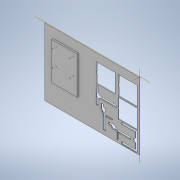
# Autodesk Inventor part: Base
Saved by Autodesk Inventor 2022 (Build 260153000, 153)
## iProperties
Created: 2022-11-21
Part Number: Base
Material: Genérico
Document SubType Name: Modeling
Designer: javie
Density: 1 g/cm^3
Appearance: Valor por defecto
Autodesk Inventor part; units mm, degrees
ref_plane "YZ Plane" through (0, 0, 0) normal (1, 0, 0) x (0, 1, 0)
ref_plane "XZ Plane" through (0, 0, 0) normal (0, 1, 0) x (-1, 0, 0)
ref_plane "XY Plane" through (0, 0, 0) normal (0, 0, 1) x (1, 0, 0)
sketch "Boceto1" plane through (0, 0, 0) normal (0, 0, 1) x (1, 0, 0)
  circle A0 centre (-147.8951, -213.4011) radius 3.5
  circle A1 centre (-21.8951, -213.4011) radius 3.5
  circle A2 centre (-147.8951, -339.4011) radius 3.5
  circle A3 centre (-21.8951, -339.4011) radius 3.5
  circle A4 centre (-309.6354, -191.7984) radius 3.5
  circle A5 centre (-309.6354, -65.7984) radius 3.5
  circle A6 centre (-183.6354, -191.7984) radius 3.5
  circle A7 centre (-183.6354, -65.7984) radius 3.5
  circle A8 centre (-146.8282, -191.7984) radius 3.5
  circle A9 centre (-146.8282, -65.7984) radius 3.5
  circle A10 centre (-20.8282, -191.7984) radius 3.5
  circle A11 centre (-20.8282, -65.7984) radius 3.5
  circle A12 centre (-217.6796, -404.2586) radius 3.5
  circle A13 centre (-276.1451, -313.6219) radius 3.5
  line L0 (-317.237, -262.6146) -> (-317.237, -210.942)
  line L1 (-317.237, -210.942) -> (-302.237, -210.942)
  line L2 (-302.237, -210.942) -> (-302.237, -256.0675)
  circle A14 centre (-309.9844, -222.642) radius 3.5
  line L3 (-29.8951, -324.021) -> (-29.8951, -338.4011)
  line L4 (-29.8951, -338.4011) -> (-139.8951, -338.4011)
  line L5 (-139.8951, -338.4011) -> (-139.8951, -324.4011)
  line L6 (-139.8951, -324.4011) -> (-139.8951, -292.2756)
  arc A15 (-157.9179, -437.9883) -> (-161.9179, -437.9883) centre (-159.9179, -437.9883) ccw
  line L7 (-157.9179, -437.9883) -> (-157.9179, -475.168)
  arc A16 (-161.9179, -475.168) -> (-157.9179, -475.168) centre (-159.9179, -475.168) ccw
  line L8 (-161.9179, -475.168) -> (-161.9179, -437.9883)
  line L9 (-61.4887, -423.9723) -> (-61.4887, -416.4723)
  line L10 (-61.4887, -416.4723) -> (-145.4587, -416.4723)
  arc A17 (-148.1709, -416.0975) -> (-145.4587, -416.4723) centre (-145.4587, -406.4723) ccw
  line L11 (-148.1709, -416.0975) -> (-172.3586, -409.282)
  arc A18 (-172.3586, -409.282) -> (-174.2641, -408.9398) centre (-175.0707, -418.9072) ccw
  arc A19 (-176.1813, -408.5942) -> (-174.2641, -408.9398) centre (-173.4575, -398.9723) ccw
  line L12 (-242.4154, -373.3836) -> (-205.2357, -373.3836)
  arc A20 (-205.2357, -373.3836) -> (-205.2357, -369.3836) centre (-205.2357, -371.3836) ccw
  line L13 (-205.2357, -369.3836) -> (-242.4154, -369.3836)
  arc A21 (-242.4154, -369.3836) -> (-242.4154, -373.3836) centre (-242.4154, -371.3836) ccw
  line L14 (-153.8282, -119.471) -> (-153.8282, -58.7984)
  line L15 (-153.8282, -58.7984) -> (-13.8282, -58.7984)
  line L16 (-13.8282, -58.7984) -> (-13.8282, -198.7984)
  line L17 (-13.8282, -198.7984) -> (-153.8282, -198.7984)
  line L18 (-153.8282, -198.7984) -> (-153.8282, -138.1258)
  line L19 (-138.8282, -144.6729) -> (-138.8282, -183.7984)
  line L20 (-138.8282, -183.7984) -> (-28.8282, -183.7984)
  line L21 (-28.8282, -183.7984) -> (-28.8282, -73.7984)
  line L22 (-28.8282, -73.7984) -> (-138.8282, -73.7984)
  line L23 (-138.8282, -73.7984) -> (-138.8282, -112.9239)
  line L24 (-316.6354, -119.471) -> (-316.6354, -58.7984)
  line L25 (-316.6354, -58.7984) -> (-176.6354, -58.7984)
  line L26 (-176.6354, -58.7984) -> (-176.6354, -198.7984)
  line L27 (-176.6354, -198.7984) -> (-316.6354, -198.7984)
  line L28 (-316.6354, -198.7984) -> (-316.6354, -138.1258)
  line L29 (-301.6354, -144.6729) -> (-301.6354, -183.7984)
  line L30 (-301.6354, -183.7984) -> (-191.6354, -183.7984)
  line L31 (-191.6354, -183.7984) -> (-191.6354, -73.7984)
  line L32 (-191.6354, -73.7984) -> (-301.6354, -73.7984)
  line L33 (-301.6354, -73.7984) -> (-301.6354, -112.9239)
  line L34 (492.5651, -223.6733) -> (492.5651, -502.5112)
  line L35 (492.5651, -502.5112) -> (302.0855, -502.5112)
  line L36 (302.0855, -502.5112) -> (302.0855, -223.6733)
  line L37 (302.0855, -223.6733) -> (492.5651, -223.6733)
  circle A22 centre (459.6774, -256.2358) radius 2.5
  circle A23 centre (459.6774, -382.2358) radius 2.5
  circle A24 centre (333.6774, -256.2358) radius 2.5
  circle A25 centre (333.6774, -382.2358) radius 2.5
  circle A26 centre (-22, -486) radius 3.5
  line L38 (-128.3631, -478) -> (-30, -478)
  line L39 (-30, -478) -> (-30, -438.8745)
  line L40 (-128.3631, -493) -> (-128.3631, -478)
  line L41 (-128.3631, -353) -> (-15, -353)
  line L42 (-15, -353) -> (-15, -413.6726)
  line L43 (-128.3631, -368) -> (-128.3631, -353)
  circle A27 centre (-22, -360) radius 3.5
  arc A28 (-316.6354, -119.471) -> (-316.6354, -138.1258) centre (-303.6354, -128.7984) ccw
  arc A29 (-153.8282, -119.471) -> (-153.8282, -138.1258) centre (-140.8282, -128.7984) ccw
  arc A30 (-317.237, -262.6146) -> (-317.237, -281.2693) centre (-304.237, -271.942) ccw
  arc A31 (-154.8951, -267.0738) -> (-154.8951, -285.7285) centre (-141.8951, -276.4011) ccw
  arc A32 (-281.1451, -332.0528) -> (-271.8095, -355.1202) centre (-267.1529, -339.8128) ccw
  arc A33 (-30, -407.1255) -> (-30, -438.8745) centre (-28, -423) ccw
  arc A34 (-207.2589, -415.9528) -> (-179.6123, -423.9723) centre (-191.4887, -413.2508) ccw
  arc A35 (-301.6354, -144.6729) -> (-301.6354, -112.9239) centre (-303.6354, -128.7984) ccw
  arc A36 (-138.8282, -144.6729) -> (-138.8282, -112.9239) centre (-140.8282, -128.7984) ccw
  line L44 (-281.1451, -332.0528) -> (-281.1451, -306.6219)
  line L45 (-281.1451, -306.6219) -> (-266.151, -306.6219)
  line L46 (-266.151, -306.6219) -> (-266.151, -318.4649)
  arc A37 (-266.151, -318.4649) -> (-264.4509, -324.0426) centre (-256.151, -318.4649) ccw
  line L47 (-256.4313, -351.6892) -> (-256.4313, -356.4621)
  arc A38 (-256.4313, -356.4621) -> (-256.0565, -359.1742) centre (-246.4313, -356.4621) ccw
  line L48 (-256.0565, -359.1742) -> (-253.7433, -367.3836)
  line L49 (-253.7433, -367.3836) -> (-201.7433, -367.3836)
  arc A39 (-201.7433, -375.3836) -> (-201.7433, -367.3836) centre (-201.4872, -371.3836) ccw
  line L50 (-201.7433, -375.3836) -> (-251.4891, -375.3836)
  line L51 (-251.4891, -375.3836) -> (-249.3062, -383.1307)
  arc A40 (-248.9313, -385.8428) -> (-249.3062, -383.1307) centre (-258.9313, -385.8428) ccw
  line L52 (-248.9313, -385.8428) -> (-248.9313, -469.8128)
  line L53 (-248.9313, -469.8128) -> (-263.9313, -469.8128)
  line L54 (-263.9313, -469.8128) -> (-263.9313, -385.8428)
  arc A41 (-263.9313, -385.8428) -> (-264.3062, -383.1307) centre (-273.9313, -385.8428) ccw
  line L55 (-264.3062, -383.1307) -> (-271.1217, -358.943)
  arc A42 (-271.4639, -357.0374) -> (-271.1217, -358.943) centre (-261.4965, -356.2308) ccw
  arc A43 (-271.4639, -357.0374) -> (-271.8095, -355.1202) centre (-281.4313, -357.8441) ccw
  arc A44 (-256.4313, -351.6892) -> (-264.4509, -324.0426) centre (-267.1529, -339.8128) ccw
  line L56 (-139.8951, -260.5266) -> (-139.8951, -214.4011)
  line L57 (-139.8951, -214.4011) -> (-29.8951, -214.4011)
  line L58 (-29.8951, -214.4011) -> (-29.8951, -267.9011)
  line L59 (-29.8951, -267.9011) -> (-14.8951, -267.9011)
  line L60 (-14.8951, -267.9011) -> (-14.8951, -206.4011)
  line L61 (-14.8951, -206.4011) -> (-154.8951, -206.4011)
  line L62 (-154.8951, -206.4011) -> (-154.8951, -267.0738)
  line L63 (-154.8951, -285.7285) -> (-154.8951, -346.4011)
  line L64 (-154.8951, -346.4011) -> (-14.8951, -346.4011)
  line L65 (-14.8951, -346.4011) -> (-14.8951, -284.9011)
  line L66 (-14.8951, -284.9011) -> (-29.8951, -284.9011)
  line L67 (-29.8951, -284.9011) -> (-29.8951, -324.4011)
  arc A45 (-139.8951, -292.2756) -> (-139.8951, -260.5266) centre (-141.8951, -276.4011) ccw
  line L68 (-290.1037, -264.442) -> (-167.237, -264.442)
  line L69 (-167.237, -264.442) -> (-167.237, -279.442)
  line L70 (-167.237, -279.442) -> (-290.1037, -279.442)
  line L71 (-302.237, -287.8165) -> (-302.237, -332.942)
  line L72 (-302.237, -332.942) -> (-317.237, -332.942)
  line L73 (-317.237, -332.942) -> (-317.237, -281.2693)
  arc A46 (-302.237, -287.8165) -> (-290.1037, -279.442) centre (-304.237, -271.942) ccw
  arc A47 (-290.1037, -264.442) -> (-302.237, -256.0675) centre (-304.237, -271.942) ccw
  line L74 (-15, -432.3274) -> (-15, -493)
  line L75 (-15, -493) -> (-128.3631, -493)
  line L76 (-30, -407.1255) -> (-30, -368)
  line L77 (-30, -368) -> (-128.3631, -368)
  arc A48 (-15, -432.3274) -> (-15, -413.6726) centre (-28, -423) ccw
  line L78 (-179.6123, -423.9723) -> (-174.8394, -423.9723)
  arc A49 (-172.1273, -424.3472) -> (-174.8394, -423.9723) centre (-174.8394, -433.9723) ccw
  line L79 (-172.1273, -424.3472) -> (-163.9179, -426.6604)
  line L80 (-163.9179, -426.6604) -> (-163.9179, -478.6604)
  arc A50 (-163.9179, -478.6604) -> (-155.9179, -478.6604) centre (-159.9179, -478.9165) ccw
  line L81 (-155.9179, -478.6604) -> (-155.9179, -428.9146)
  line L82 (-155.9179, -428.9146) -> (-148.1709, -431.0975)
  arc A51 (-148.1709, -431.0975) -> (-145.4587, -431.4723) centre (-145.4587, -421.4723) ccw
  line L83 (-145.4587, -431.4723) -> (-61.4887, -431.4723)
  line L84 (-61.4887, -431.4723) -> (-61.4887, -416.4723)
  line L85 (-199.2488, -399.2586) -> (-224.6796, -399.2586)
  line L86 (-224.6796, -399.2586) -> (-224.6796, -414.2527)
  line L87 (-224.6796, -414.2527) -> (-212.8366, -414.2527)
  arc A52 (-207.2589, -415.9528) -> (-212.8366, -414.2527) centre (-212.8366, -424.2527) ccw
  arc A53 (-176.1813, -408.5942) -> (-199.2488, -399.2586) centre (-191.4887, -413.2508) ccw
  line L88 (-29.8951, -267.9011) -> (-29.8951, -284.9011)
  line L89 (-14.8951, -267.9011) -> (-14.8951, -284.9011)
  line L90 (0, 0) -> (-700, 0)
  line L91 (-700, 0) -> (-700, -500)
  line L92 (-700, -500) -> (0, -500)
  line L93 (0, -500) -> (0, 0)
  point P0 (0, -463)
  point P1 (332, -463)
  point P2 (332, 0)
  point P3 (50.8356, -262.3941)
  point P4 (65.8296, -262.3941)
  point P5 (65.8296, -274.2371)
  point P6 (67.5297, -279.8148)
  point P7 (75.5493, -307.4614)
  point P8 (75.5493, -312.2343)
  point P9 (75.9241, -314.9465)
  point P10 (78.2373, -323.1558)
  point P11 (130.2373, -323.1558)
  point P12 (130.2373, -331.1558)
  point P13 (80.4915, -331.1558)
  point P14 (82.6745, -338.9029)
  point P15 (83.0493, -341.615)
  point P16 (83.0493, -425.585)
  point P17 (68.0493, -425.585)
  point P18 (68.0493, -341.615)
  point P19 (67.6745, -338.9029)
  point P20 (60.8589, -314.7152)
  point P21 (60.5167, -312.8096)
  point P22 (60.1712, -310.8924)
  point P23 (50.8356, -287.825)
  point P24 (316.9806, -388.0996)
  point P25 (316.9806, -448.7722)
  point P26 (203.6175, -448.7722)
  point P27 (203.6175, -433.7722)
  point P28 (301.9806, -433.7722)
  point P29 (301.9806, -394.6467)
  point P30 (301.9806, -362.8977)
  point P31 (301.9806, -323.7722)
  point P32 (203.6175, -323.7722)
  point P33 (203.6175, -308.7722)
  point P34 (316.9806, -308.7722)
  point P35 (316.9806, -369.4448)
  point P36 (15.3452, -75.2432)
  point P37 (15.3452, -14.5706)
  point P38 (155.3452, -14.5706)
  point P39 (155.3452, -154.5706)
  point P40 (15.3452, -154.5706)
  point P41 (15.3452, -93.898)
  point P42 (178.1524, -75.2432)
  point P43 (178.1524, -14.5706)
  point P44 (318.1524, -14.5706)
  point P45 (318.1524, -154.5706)
  point P46 (178.1524, -154.5706)
  point P47 (178.1524, -93.898)
  point P48 (29.7436, -243.5887)
  point P49 (29.7436, -288.7142)
  point P50 (14.7436, -288.7142)
  point P51 (14.7436, -237.0415)
  point P52 (14.7436, -218.3868)
  point P53 (14.7436, -166.7142)
  point P54 (29.7436, -166.7142)
  point P55 (29.7436, -211.8397)
  point P56 (41.8769, -220.2142)
  point P57 (164.7436, -220.2142)
  point P58 (164.7436, -235.2142)
  point P59 (41.8769, -235.2142)
  point P60 (186.5219, -372.2445)
  point P61 (270.4919, -372.2445)
  point P62 (270.4919, -379.7445)
  point P63 (270.4919, -387.2445)
  point P64 (186.5219, -387.2445)
  point P65 (183.8098, -386.8697)
  point P66 (176.0627, -384.6868)
  point P67 (176.0627, -434.4326)
  point P68 (168.0627, -434.4326)
  point P69 (168.0627, -382.4326)
  point P70 (159.8533, -380.1194)
  point P71 (157.1412, -379.7445)
  point P72 (152.3683, -379.7445)
  point P73 (124.7217, -371.725)
  point P74 (119.144, -370.0249)
  point P75 (107.301, -370.0249)
  point P76 (107.301, -355.0308)
  point P77 (132.7318, -355.0308)
  point P78 (155.7993, -364.3664)
  point P79 (157.7165, -364.712)
  point P80 (159.622, -365.0542)
  point P81 (183.8098, -371.8697)
  point P82 (317.0855, -240.6733)
  point P83 (317.0855, -302.1733)
  point P84 (177.0855, -302.1733)
  point P85 (177.0855, -241.5007)
  point P86 (177.0855, -222.846)
  point P87 (177.0855, -162.1733)
  point P88 (317.0855, -162.1733)
  point P89 (317.0855, -223.6733)
  point P90 (-271.8095, -355.1202)
  point P91 (-281.1451, -332.0528)
  point P92 (-317.237, -281.2693)
  point P93 (-145.4587, -431.4723)
  point P94 (-155.9179, -478.6604)
  point P95 (-172.1273, -424.3472)
  point P96 (-179.6123, -423.9723)
  point P97 (-207.2589, -415.9528)
  point P98 (-148.1709, -416.0975)
  dimension "d10" = 700
  dimension "d11" = 500
  constraints: 188 end point, 66 point on circle, 54 centre point, 2 parallel, 1 horizontal, 1 perpendicular
  measures "d10" distance of L92.end L91.end
  measures "d11" distance of L91.end L90.end
extrude "Extrusión2" add sketch "Boceto1" along normal blind 5 contours L93 L92 L91 L90
sketch "Boceto3" plane through (0, 0, 5) normal (0, 0, 1) x (1, 0, 0)
  line L0 (-449.5205, -71.1621) -> (-449.5205, -350)
  line L1 (-449.5205, -350) -> (-640, -350)
  line L2 (-640, -350) -> (-640, -71.1621)
  line L3 (-640, -71.1621) -> (-449.5205, -71.1621)
  circle A0 centre (-482.4081, -103.7246) radius 2.5
  circle A1 centre (-482.4081, -229.7246) radius 2.5
  circle A2 centre (-608.4081, -103.7246) radius 2.5
  circle A3 centre (-608.4081, -229.7246) radius 2.5
  line L4 (0, 0) -> (-700, 0)
  line L5 (-700, 0) -> (-700, -500)
  line L6 (-700, -500) -> (0, -500)
  line L7 (0, -500) -> (0, 0)
  point P0 (0, -463)
  point P1 (332, -463)
  point P2 (332, 0)
  point P3 (50.8356, -262.3941)
  point P4 (65.8296, -262.3941)
  point P5 (65.8296, -274.2371)
  point P6 (67.5297, -279.8148)
  point P7 (75.5493, -307.4614)
  point P8 (75.5493, -312.2343)
  point P9 (75.9241, -314.9465)
  point P10 (78.2373, -323.1558)
  point P11 (130.2373, -323.1558)
  point P12 (130.2373, -331.1558)
  point P13 (80.4915, -331.1558)
  point P14 (82.6745, -338.9029)
  point P15 (83.0493, -341.615)
  point P16 (83.0493, -425.585)
  point P17 (68.0493, -425.585)
  point P18 (68.0493, -341.615)
  point P19 (67.6745, -338.9029)
  point P20 (60.8589, -314.7152)
  point P21 (60.5167, -312.8096)
  point P22 (60.1712, -310.8924)
  point P23 (50.8356, -287.825)
  point P24 (316.9806, -388.0996)
  point P25 (316.9806, -448.7722)
  point P26 (203.6175, -448.7722)
  point P27 (203.6175, -433.7722)
  point P28 (301.9806, -433.7722)
  point P29 (301.9806, -394.6467)
  point P30 (301.9806, -362.8977)
  point P31 (301.9806, -323.7722)
  point P32 (203.6175, -323.7722)
  point P33 (203.6175, -308.7722)
  point P34 (316.9806, -308.7722)
  point P35 (316.9806, -369.4448)
  point P36 (15.3452, -75.2432)
  point P37 (15.3452, -14.5706)
  point P38 (155.3452, -14.5706)
  point P39 (155.3452, -154.5706)
  point P40 (15.3452, -154.5706)
  point P41 (15.3452, -93.898)
  point P42 (178.1524, -75.2432)
  point P43 (178.1524, -14.5706)
  point P44 (318.1524, -14.5706)
  point P45 (318.1524, -154.5706)
  point P46 (178.1524, -154.5706)
  point P47 (178.1524, -93.898)
  point P48 (29.7436, -243.5887)
  point P49 (29.7436, -288.7142)
  point P50 (14.7436, -288.7142)
  point P51 (14.7436, -237.0415)
  point P52 (14.7436, -218.3868)
  point P53 (14.7436, -166.7142)
  point P54 (29.7436, -166.7142)
  point P55 (29.7436, -211.8397)
  point P56 (41.8769, -220.2142)
  point P57 (164.7436, -220.2142)
  point P58 (164.7436, -235.2142)
  point P59 (41.8769, -235.2142)
  point P60 (186.5219, -372.2445)
  point P61 (270.4919, -372.2445)
  point P62 (270.4919, -379.7445)
  point P63 (270.4919, -387.2445)
  point P64 (186.5219, -387.2445)
  point P65 (183.8098, -386.8697)
  point P66 (176.0627, -384.6868)
  point P67 (176.0627, -434.4326)
  point P68 (168.0627, -434.4326)
  point P69 (168.0627, -382.4326)
  point P70 (159.8533, -380.1194)
  point P71 (157.1412, -379.7445)
  point P72 (152.3683, -379.7445)
  point P73 (124.7217, -371.725)
  point P74 (119.144, -370.0249)
  point P75 (107.301, -370.0249)
  point P76 (107.301, -355.0308)
  point P77 (132.7318, -355.0308)
  point P78 (155.7993, -364.3664)
  point P79 (157.7165, -364.712)
  point P80 (159.622, -365.0542)
  point P81 (183.8098, -371.8697)
  point P82 (317.0855, -240.6733)
  point P83 (317.0855, -302.1733)
  point P84 (177.0855, -302.1733)
  point P85 (177.0855, -241.5007)
  point P86 (177.0855, -222.846)
  point P87 (177.0855, -162.1733)
  point P88 (317.0855, -162.1733)
  point P89 (317.0855, -223.6733)
  point P90 (-281.1451, -306.6219)
  point P91 (-266.151, -306.6219)
  point P92 (-266.151, -318.4649)
  point P93 (-264.4509, -324.0426)
  point P94 (-256.4313, -351.6892)
  point P95 (-256.4313, -356.4621)
  point P96 (-256.0565, -359.1742)
  point P97 (-253.7433, -367.3836)
  point P98 (-201.7433, -367.3836)
  point P99 (-201.7433, -375.3836)
  point P100 (-251.4891, -375.3836)
  point P101 (-249.3062, -383.1307)
  point P102 (-248.9313, -385.8428)
  point P103 (-248.9313, -469.8128)
  point P104 (-263.9313, -469.8128)
  point P105 (-263.9313, -385.8428)
  point P106 (-264.3062, -383.1307)
  point P107 (-271.1217, -358.943)
  point P108 (-271.4639, -357.0374)
  point P109 (-271.8095, -355.1202)
  point P110 (-281.1451, -332.0528)
  point P111 (-15, -432.3274)
  point P112 (-15, -493)
  point P113 (-128.3631, -493)
  point P114 (-128.3631, -478)
  point P115 (-30, -478)
  point P116 (-30, -438.8745)
  point P117 (-30, -407.1255)
  point P118 (-30, -368)
  point P119 (-128.3631, -368)
  point P120 (-128.3631, -353)
  point P121 (-15, -353)
  point P122 (-15, -413.6726)
  point P123 (-316.6354, -119.471)
  point P124 (-316.6354, -58.7984)
  point P125 (-176.6354, -58.7984)
  point P126 (-176.6354, -198.7984)
  point P127 (-316.6354, -198.7984)
  point P128 (-316.6354, -138.1258)
  point P129 (-153.8282, -119.471)
  point P130 (-153.8282, -58.7984)
  point P131 (-13.8282, -58.7984)
  point P132 (-13.8282, -198.7984)
  point P133 (-153.8282, -198.7984)
  point P134 (-153.8282, -138.1258)
  point P135 (-302.237, -287.8165)
  point P136 (-302.237, -332.942)
  point P137 (-317.237, -332.942)
  point P138 (-317.237, -281.2693)
  point P139 (-317.237, -262.6146)
  point P140 (-317.237, -210.942)
  point P141 (-302.237, -210.942)
  point P142 (-302.237, -256.0675)
  point P143 (-290.1037, -264.442)
  point P144 (-167.237, -264.442)
  point P145 (-167.237, -279.442)
  point P146 (-290.1037, -279.442)
  point P147 (-145.4587, -416.4723)
  point P148 (-61.4887, -416.4723)
  point P149 (-61.4887, -423.9723)
  point P150 (-61.4887, -431.4723)
  point P151 (-145.4587, -431.4723)
  point P152 (-148.1709, -431.0975)
  point P153 (-155.9179, -428.9146)
  point P154 (-155.9179, -478.6604)
  point P155 (-163.9179, -478.6604)
  point P156 (-163.9179, -426.6604)
  point P157 (-172.1273, -424.3472)
  point P158 (-174.8394, -423.9723)
  point P159 (-179.6123, -423.9723)
  point P160 (-207.2589, -415.9528)
  point P161 (-212.8366, -414.2527)
  point P162 (-224.6796, -414.2527)
  point P163 (-224.6796, -399.2586)
  point P164 (-199.2488, -399.2586)
  point P165 (-176.1813, -408.5942)
  point P166 (-174.2641, -408.9398)
  point P167 (-172.3586, -409.282)
  point P168 (-148.1709, -416.0975)
  point P169 (-14.8951, -284.9011)
  point P170 (-14.8951, -346.4011)
  point P171 (-154.8951, -346.4011)
  point P172 (-154.8951, -285.7285)
  point P173 (-154.8951, -267.0738)
  point P174 (-154.8951, -206.4011)
  point P175 (-14.8951, -206.4011)
  point P176 (-14.8951, -267.9011)
  dimension "d14" = 700
  dimension "d15" = 500
  dimension "d16" = 60
  dimension "d18" = 150
  constraints: 16 end point, 4 centre point, 2 parallel, 1 horizontal, 1 perpendicular
  measures "d14" distance of L6.end L5.end
  measures "d15" distance of L5.end L4.end
  measures "d16" distance from line of point (-640, -350) L5
  measures "d18" distance between parallel lines of L6 L1
extrude "Extrusión3" add sketch "Boceto3" along normal blind 9 contours L0 L1 L2 L3
sketch "Boceto4" plane through (0, 0, 14) normal (0, 0, 1) x (1, 0, 0)
  circle A0 centre (-608.4081, -103.7246) radius 2.5 projected
  circle A1 centre (-608.4081, -103.7246) radius 2.5
  circle A2 centre (-482.4081, -103.7246) radius 2.5 projected
  circle A3 centre (-482.4081, -103.7246) radius 2.5
  circle A4 centre (-608.4081, -229.7246) radius 2.5 projected
  circle A5 centre (-608.4081, -229.7246) radius 2.5
  circle A6 centre (-482.4081, -229.7246) radius 2.5
  point P0 (0, 0)
  dimension "d21" = 5
  constraints: 4 centre point, 3 coincident
  measures "d21" diameter of A6
extrude "Extrusión4" add sketch "Boceto4" along normal blind 25
